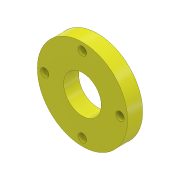
# Autodesk Inventor part: ground_support_3
Saved by Autodesk Inventor 2018 (Build 220112000, 112)
## iProperties
Created: 2019-12-28
Part Number: ground_support_3
Material: Generic
Document SubType Name: Modeling
Designer: nnico
Density: 1 g/cm^3
Appearance: Yellow
Author: nnico
Autodesk Inventor part; units mm, degrees
ref_plane "YZ Plane" through (0, 0, 0) normal (1, 0, 0) x (0, 1, 0)
ref_plane "XZ Plane" through (0, 0, 0) normal (0, 1, 0) x (-1, 0, 0)
ref_plane "XY Plane" through (0, 0, 0) normal (0, 0, 1) x (1, 0, 0)
sketch "Sketch1" plane through (0, 0, 0) normal (0, 1, 0) x (-1, 0, 0)
  circle A0 centre (0, 0) radius 15
  circle A1 centre (0, 0) radius 6.25
  dimension "d0" = 30
  dimension "d1" = 12.5
  constraints: 2 centre point, 2 coincident
  measures "d0" diameter of A0
  measures "d1" diameter of A1
extrude "Extrusion1" add sketch "Sketch1" along normal blind 5
sketch "Sketch2" plane through (0, 5, 0) normal (0, 1, 0) x (1, 0, 0)
  line L0 (0, 0) -> (0, 15) construction
  circle A0 centre (0, 0) radius 15 construction
  circle A1 centre (0, 0) radius 12.5 construction
  line L1 (-12.5, 0) -> (0, 12.5) construction
  line L2 (0, 12.5) -> (12.5, 0) construction
  line L3 (12.5, 0) -> (0, -12.5) construction
  line L4 (0, -12.5) -> (-12.5, 0) construction
  line L5 (0, 0) -> (-15, 0) construction
  circle A2 centre (0, 12.5) radius 1.375
  circle A3 centre (-12.5, 0) radius 1.375
  circle A4 centre (0, -12.5) radius 1.375
  circle A5 centre (12.5, 0) radius 1.375
  dimension "d4" = 25
  dimension "d5" = 2.75
  dimension "d6" = 2.75
  dimension "d7" = 2.75
  dimension "d8" = 2.75
  constraints: 12 end point, 5 centre point, 5 coincident, 5 point on circle, 2 parallel, 2 point on line, 1 horizontal, 1 perpendicular, 1 vertical
  measures "d4" diameter of A1
  measures "d5" diameter of A2
  measures "d6" diameter of A3
  measures "d7" diameter of A4
  measures "d8" diameter of A5
extrude "Extrusion2" cut sketch "Sketch2" against normal blind 5
body "Solid1"
